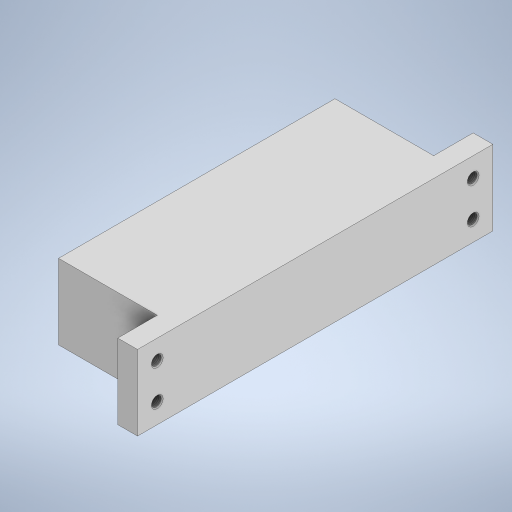
# Autodesk Inventor part: Подставка подшипника
Saved by Autodesk Inventor 2023 (Build 270158000, 158)
## iProperties
Created: 2022-05-17
Part Number: Подставка подшипника
Material: Типовые
Document SubType Name: Modeling
Designer: avkap
Density: 1 g/cm^3
Appearance: По умолчанию
Author: avkap
Autodesk Inventor part; units mm, degrees
ref_plane "YZ Plane" through (0, 0, 0) normal (1, 0, 0) x (0, 1, 0)
ref_plane "XZ Plane" through (0, 0, 0) normal (0, 1, 0) x (-1, 0, 0)
ref_plane "XY Plane" through (0, 0, 0) normal (0, 0, 1) x (1, 0, 0)
sketch "Эскиз1" plane through (0, 0, 0) normal (0, 1, 0) x (-1, 0, 0)
  line L0 (0, 0) -> (10, 0)
  line L1 (10, 0) -> (10, -20)
  line L2 (10, -20) -> (60, -20)
  line L3 (60, -20) -> (60, -160)
  line L4 (60, -160) -> (10, -160)
  line L5 (10, -160) -> (10, -180)
  line L6 (10, -180) -> (0, -180)
  line L7 (0, -180) -> (0, 0)
  dimension "d0" = 10
  dimension "d1" = 20
  dimension "d2" = 50
  dimension "d3" = 140
  dimension "d4" = 20
  constraints: 16 end point, 6 perpendicular, 2 point on line, 1 horizontal
  measures "d0" distance of L0.start L0.end
  measures "d1" distance of L0.end L1.end
  measures "d2" distance of L1.end L2.end
  measures "d3" distance of L2.end L3.end
  measures "d4" distance of L4.end L5.end
extrude "Выдавливание1" add sketch "Эскиз1" along normal blind 38
sketch "Эскиз2" plane through (-10, 0, -20) normal (-1, 0, 0) x (0, 0, 1)
  line L0 (0, 0) -> (20, 0) projected
  line L1 (20, 0) -> (0, 0)
  line L2 (0, 0) -> (10, 0)
  line L3 (10, 0) -> (10, 10)
  line L4 (20, 38) -> (-160, 38) projected
  line L5 (10, 38) -> (10, 28)
  line L6 (-140, 0) -> (-140, 38) projected
  line L7 (-160, 38) -> (-140, 38)
  line L8 (-140, 38) -> (-150, 38)
  line L9 (-150, 38) -> (-150, 28)
  line L10 (-150, 0) -> (-150, 10)
  circle A0 centre (10, 10) radius 2.5
  circle A1 centre (10, 28) radius 2.5
  circle A2 centre (-150, 10) radius 2.5
  circle A3 centre (-150, 28) radius 2.5
  dimension "d7" = 10
  dimension "d8" = 10
  dimension "d9" = 10
  dimension "d10" = 10
  dimension "d11" = 5
  dimension "d12" = 5
  dimension "d13" = 5
  dimension "d14" = 5
  constraints: 16 end point, 6 point on line, 4 centre point, 4 coincident, 3 perpendicular, 2 midpoint, 1 horizontal
  measures "d7" distance of L2.end L3.end
  measures "d8" distance of L5.start L5.end
  measures "d9" distance of L8.end L9.end
  measures "d10" distance of L10.start L10.end
  measures "d11" diameter of A0
  measures "d12" diameter of A1
  measures "d13" diameter of A2
  measures "d14" diameter of A3
extrude "Выдавливание2" cut sketch "Эскиз2" against normal blind 44.25
thread "Резьба1" size "M5x0.8" class "6H" standard "ISO Metric profile" full length
thread "Резьба2" size "M5x0.8" class "6H" standard "ISO Metric profile" full length
thread "Резьба3" size "M5x0.8" class "6H" standard "ANSI Metric M Profile" full length
thread "Резьба4" size "M5x0.8" class "6H" standard "ANSI Metric M Profile" full length
chamfer "Фаска1" distance 0.5 angle 45 8 edges at (-10, 10, -12.5) (-10, 28, -12.5) (-10, 10, -172.5) (-10, 28, -172.5) (0, 28, -172.5) (0, 10, -172.5) (0, 10, -12.5) (0, 28, -12.5)
sketch "Эскиз3" plane through (-60, 0, -160) normal (-1, 0, 0) x (0, 0, 1)
  line L0 (140, 0) -> (140, 38) projected
  line L1 (140, 0) -> (140, 19)
  line L2 (140, 0) -> (70, 0)
  line L3 (160, 0) -> (-20, 0) projected
  line L4 (70, 20) -> (122.5, 20)
  line L5 (122.5, 20) -> (17.5, 20)
  line L6 (70, 20) -> (70, 0)
  circle A0 centre (122.5, 20) radius 6
  circle A1 centre (17.5, 20) radius 6
  dimension "d28" = 52.5
  dimension "d29" = 105
  dimension "d30" = 12
  dimension "d31" = 12
  constraints: 10 end point, 2 centre point, 2 coincident, 2 horizontal, 2 midpoint, 1 perpendicular
  measures "d28" distance of L4.start L4.end
  measures "d29" distance of L4.end L5.end
  measures "d30" diameter of A0
  measures "d31" diameter of A1
extrude "Выдавливание3" cut sketch "Эскиз3" against normal blind 20
chamfer "Фаска2" distance 0.5 angle 45 2 edges at (-60, 20, -43.5) (-60, 20, -148.5)
thread "Резьба5" size "M12x1.75" class "6H" standard "ANSI Metric M Profile" full length
thread "Резьба6" size "M12x1.75" class "6H" standard "ANSI Metric M Profile" full length
